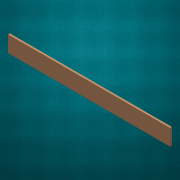
# Autodesk Inventor part: Bed Rail
Saved by Autodesk Inventor 2017 (Build 210142000, 142)
## iProperties
Created: 2017-06-03
Part Number: Bed Rail
Material: Wood (Cherry)
Document SubType Name: Modeling
Designer: Michael
Density: 0.63 g/cm^3
Appearance: Cherry - Natural Low Gloss
Author: Michael
Autodesk Inventor part; units mm, degrees
ref_plane "YZ Plane" through (0, 0, 0) normal (1, 0, 0) x (0, 1, 0)
ref_plane "XZ Plane" through (0, 0, 0) normal (0, 1, 0) x (-1, 0, 0)
ref_plane "XY Plane" through (0, 0, 0) normal (0, 0, 1) x (1, 0, 0)
sketch "Sketch1" plane through (0, 0, 0) normal (1, 0, 0) x (0, 1, 0)
  line L0 (-101.6, 11.1125) -> (101.6, 11.1125)
  line L1 (101.6, 11.1125) -> (101.6, -11.1125)
  line L2 (101.6, -11.1125) -> (-101.6, -11.1125)
  line L3 (-101.6, -11.1125) -> (-101.6, 11.1125)
  line L4 (-101.6, 11.1125) -> (101.6, -11.1125) construction
  line L5 (101.6, 11.1125) -> (-101.6, -11.1125) construction
  point P0 (0, 0)
  dimension "d0" = 22.225
  dimension "d1" = 203.2
  constraints: 12 end point, 2 midpoint, 2 parallel, 1 horizontal, 1 perpendicular
  measures "d0" distance of L0.end L1.end
  measures "d1" distance of L0.start L0.end
extrude "Extrusion1" add sketch "Sketch1" along normal mid plane 2028.825
body "Solid1"
